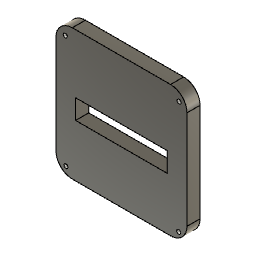
_tampa da caixinha Morea.98c9afd8-4004-429a-9e04-4d437f5e4602 (Autodesk Fusion 360 design; units mm, degrees)
Autodesk Fusion 360 part; units mm, degrees
box "Primitiva de caixa1" add length 200 width 200 height 20 placed x (0, 0, 1) y (1, 0, 0) z (0, 1, 0) at (0, 0, 0)
fillet "Arredondamento1" radius 25 4 edges at (0, 10, 200) (0, 10, 0) (200, 10, 0) (200, 10, 200)
box "Primitiva de caixa2" add length 20 width 130 height 10 placed x (0, 0, 1) y (-1, 0, 0) z (0, -1, 0) at (170, 0, 50)
delete_face "Excluir face1" 1 faces at (83.3333, -3.3333, 70)
sketch "Esboço4" plane through (0, 0, 0) normal (0, -1, 0) x (1, 0, 0)
  line L0 (175, 200) -> (25, 200)
  arc A0 (25, 200) -> (0, 175) centre (25, 175) ccw
  line L1 (0, 175) -> (0, 25)
  arc A1 (0, 25) -> (25, 0) centre (25, 25) ccw
  line L2 (25, 0) -> (175, 0)
  arc A2 (175, 0) -> (200, 25) centre (175, 25) ccw
  line L3 (200, 25) -> (200, 175)
  arc A3 (200, 175) -> (175, 200) centre (175, 175) ccw
  line L4 (30, 110) -> (170, 110)
  line L5 (170, 110) -> (170, 80)
  line L6 (170, 80) -> (30, 80)
  line L7 (30, 80) -> (30, 110)
  constraint horizontal L4
  constraint vertical L5
  constraint horizontal L6
  constraint vertical L7
extrude "Extrusão1" cut sketch "Esboço4" against normal blind 60 contours L4 L5 L6 L7
hole "Furo1" at (25, 0, 175) direction (0, 1, 0) diameter 7 depth 30 tip angle 118
move_face "MoveFace1" to x (1, 0, 0) y (0, 1, 0) z (0, 0, 1) at (-10, 0, 0) 1 faces at (26.1971, 6.6667, 178.2889)
move_face "MoveFace2" to x (1, 0, 0) y (0, 1, 0) z (0, 0, 1) at (-1.4138, 0, 8.7744) 1 faces at (16.1971, 6.6667, 178.2889)
thread "Rosca1" "ISO Metric profile 7.0 M7x1 6H" major diameter 7.1472 minor diameter 6.0355 pitch 1 angle 60 resizes the face on face at (11.0807, 6.6667, 186.2183)
move_face "MoveFace3" to x (1, 0, 0) y (0, 1, 0) z (0, 0, 1) at (0.6973, 0.1087, 0.5211) 1 faces at (10.6813, 6.6667, 182.9571)
hole "Furo2" at (187.9499, 0, 185.6628) direction (0, 1, 0) diameter 7 depth 30 tip angle 118
thread "Rosca2" "ISO Metric profile 7.0 M7x1 6H" major diameter 7.1472 minor diameter 6.0355 pitch 1 angle 60 resizes the face on face at (185.8365, 6.6667, 182.8728)
move_face "MoveFace4" to x (1, 0, 0) y (0, 1, 0) z (0, 0, 1) at (-0.0079, -0.2012, -0.7717) 1 faces at (186.1277, 6.6667, 183.2572)
move_face "MoveFace5" to x (1, 0, 0) y (0, 1, 0) z (0, 0, 1) at (-0.0109, -0.2777, -1.0648) 1 faces at (189.7641, 13.3333, 187.2966)
hole "Furo3" at (187.4356, 0, 11.328) direction (0, 1, 0) diameter 7 depth 30 tip angle 118
thread "Rosca3" "ISO Metric profile 7.0 M7x1 6H" major diameter 7.1472 minor diameter 6.0355 pitch 1 angle 60 resizes the face on face at (186.2386, 6.6667, 14.617)
hole "Furo4" at (15.4818, 0, 11.3605) direction (0, 1, 0) diameter 7 depth 30 tip angle 118
thread "Rosca4" "ISO Metric profile 7.0 M7x1 6H" major diameter 7.1472 minor diameter 6.0355 pitch 1 angle 60 resizes the face on face at (15.6563, 6.6667, 7.8648)
move_face "MoveFace6" to x (1, 0, 0) y (0, 1, 0) z (0, 0, 1) at (1.1869, 0.0531, 0.3818) 1 faces at (15.6322, 6.6667, 8.3465)
move_face "MoveFace7" to x (1, 0, 0) y (0, 1, 0) z (0, 0, 1) at (-1.2984, 0.1608, 0.4205) 1 faces at (16.3682, 13.3333, 8.7396)
